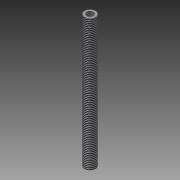
# Autodesk Inventor part: EEThreadedRod
Saved by Autodesk Inventor 2015 (Build 190159000, 159)
## iProperties
Created: 2017-01-13
Part Number: EEThreadedRod
Material: Generic
Document SubType Name: Modeling
Designer: 1esh9
Density: 1 g/cm^3
Appearance: Default
Author: 1esh9
Autodesk Inventor part; units mm, degrees
ref_plane "YZ Plane" through (0, 0, 0) normal (1, 0, 0) x (0, 1, 0)
ref_plane "XZ Plane" through (0, 0, 0) normal (0, 1, 0) x (-1, 0, 0)
ref_plane "XY Plane" through (0, 0, 0) normal (0, 0, 1) x (1, 0, 0)
sketch "Sketch1" plane through (0, 0, 0) normal (0, 0, 1) x (1, 0, 0)
  circle A0 centre (0, 0) radius 4.435
  dimension "d0" = 8.87
  constraints: 1 centre point, 1 coincident
  measures "d0" diameter of A0
extrude "Extrusion1" add sketch "Sketch1" along normal blind 108
thread "Thread1" size "M9x1.25" class "6g" standard "ANSI Metric M Profile" full length
sketch "Sketch2" plane through (0, 0, 108) normal (0, 0, 1) x (1, 0, 0)
  circle A0 centre (0, 0) radius 3
  dimension "d5" = 6
  constraints: 1 centre point, 1 coincident
  measures "d5" diameter of A0
extrude "Extrusion2" cut sketch "Sketch2" against normal blind 108
body "Solid1"
